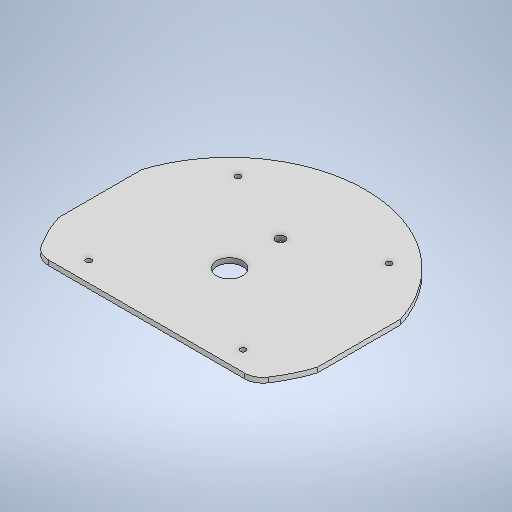
# Autodesk Inventor part: tapa_carcasa_4.0_v2
Saved by Autodesk Inventor 2025.3 (Build 293356030, 356C)
## iProperties
Created: 2025-11-26
Part Number: tapa_carcasa_4.0_v2
Material: Generic
Document SubType Name: Modeling
Designer: brene
Density: 1 g/cm^3
Appearance: Default
Author: brene
Autodesk Inventor part; units mm, degrees
ref_plane "YZ Plane" through (0, 0, 0) normal (1, 0, 0) x (0, 1, 0)
ref_plane "XZ Plane" through (0, 0, 0) normal (0, 1, 0) x (-1, 0, 0)
ref_plane "XY Plane" through (0, 0, 0) normal (0, 0, 1) x (1, 0, 0)
sketch "Sketch1" plane through (0, 0, 0) normal (0, 1, 0) x (-1, 0, 0)
  line L0 (0, 0) -> (0, 45)
  line L1 (52.9835, 45) -> (-52.9835, 45)
  line L2 (0, 0) -> (70, 0)
  line L3 (70, -22.4109) -> (70, 22.4109)
  line L4 (-70, -22.4109) -> (-70, 22.4109)
  arc A0 (70, 22.4109) -> (61.3273, 40.5118) centre (0, 0) ccw
  arc A1 (-61.3273, 40.5118) -> (-70, 22.4109) centre (0, 0) ccw
  arc A2 (-70, -22.4109) -> (70, -22.4109) centre (0, 0) ccw
  arc A3 (61.3273, 40.5118) -> (52.9835, 45) centre (52.9835, 35) ccw
  arc A4 (-52.9835, 45) -> (-61.3273, 40.5118) centre (-52.9835, 35) ccw
  point P0 (58.1141, 45)
  point P1 (-58.1141, 45)
  dimension "d33" = 45
  dimension "d34" = 58.1141
  dimension "d35" = 70
  dimension "d36" = 10
  constraints: 12 point on circle, 10 end point, 5 centre point, 4 tangent, 2 horizontal, 2 point on line, 2 symmetric about line, 2 vertical, 1 equal radius
  measures "d33" distance of L0.start L0.end
  measures "d34" distance from line of point (58.114, 45) L0
  measures "d35" distance of L0.start L2.end
  measures "d36" radius of A3
extrude "Extrusion1" add sketch "Sketch1" along normal blind 2.7
sketch "Sketch2" plane through (0, 2.7, 0) normal (0, 1, 0) x (1, 0, 0)
  circle A0 centre (0, 0) radius 7
  arc A1 (70, 22.4109) -> (-70, 22.4109) centre (0, 0) ccw projected
  line L0 (0, 0) -> (0, 73.5)
  line L1 (0, 73.5) -> (0, 27.5)
  circle A2 centre (0, 27.5) radius 2.5
  circle A3 centre (0, 0) radius 54.1913 construction
  line L2 (0, 0) -> (-67.8888, -56.0453) construction
  line L3 (0, 0) -> (-54.1913, 0)
  circle A4 centre (-41.7906, -34.5) radius 1.5
  circle A5 centre (41.7906, -34.5) radius 1.5
  circle A6 centre (0, 0) radius 61 construction
  line L4 (0, 0) -> (-40.817, 45.3318)
  circle A7 centre (-40.817, 45.3318) radius 1.5
  circle A8 centre (40.817, 45.3318) radius 1.5
  dimension "d48" = 122
  dimension "d38" = 14
  dimension "d39" = 46
  dimension "d40" = 5
  dimension "d41" = 108.3827
  dimension "d42" = 39.541
  dimension "d43" = 3
  dimension "d47" = 67.8888
  dimension "d50" = 48
  dimension "d52" = 3
  constraints: 10 end point, 7 centre point, 4 coincident, 3 point on circle, 2 point on line, 2 symmetric about line, 1 concentric, 1 horizontal, 1 vertical, 5 other
  measures "d38" diameter of A0
  measures "d39" distance of L0.end L1.end
  measures "d40" diameter of A2
  measures "d41" diameter of A3
  measures "d42" angle of L3 L2
  measures "d43" diameter of A4
  measures "d47" distance from line of L2.end L0
  measures "d50" angle of L3 L4
  measures "d52" diameter of A7
extrude "Extrusion2" cut sketch "Sketch2" against normal blind 2.7
body "Solid1"
